lower contol arm (Autodesk Fusion 360 design; units mm, degrees)
Autodesk Fusion 360 part; units mm, degrees
sketch "Sketch1" plane through (0, -20.5, 43.25) normal (0, 0, 1) x (-1, 0, 0)
  arc A0 (2.75, -18.25) -> (2.25, -17.75) centre (2.25, -18.25) ccw
  line L0 (2.25, -17.75) -> (-2.25, -17.75)
  arc A1 (-2.25, -17.75) -> (-2.75, -18.25) centre (-2.25, -18.25) ccw
  line L1 (-2.75, -18.25) -> (-2.75, -22.75)
  arc A2 (-2.75, -22.75) -> (-2.25, -23.25) centre (-2.25, -22.75) ccw
  line L2 (-2.25, -23.25) -> (2.25, -23.25)
  arc A3 (2.25, -23.25) -> (2.75, -22.75) centre (2.25, -22.75) ccw
  line L3 (2.75, -22.75) -> (2.75, -18.25)
  line L4 (2.85, -22.75) -> (2.85, -18.25)
  arc A4 (2.85, -18.25) -> (2.25, -17.65) centre (2.25, -18.25) ccw
  line L5 (2.25, -17.65) -> (-2.25, -17.65)
  arc A5 (-2.25, -17.65) -> (-2.85, -18.25) centre (-2.25, -18.25) ccw
  line L6 (-2.85, -18.25) -> (-2.85, -22.75)
  arc A6 (-2.85, -22.75) -> (-2.25, -23.35) centre (-2.25, -22.75) ccw
  line L7 (-2.25, -23.35) -> (2.25, -23.35)
  arc A7 (2.25, -23.35) -> (2.85, -22.75) centre (2.25, -22.75) ccw
  circle A8 centre (0, -20.5) radius 3.95 construction
  circle A9 centre (0, -20.5) radius 6
  line L8 (0, -20.5) -> (-20, -20.5) construction
  circle A10 centre (-20, -20.5) radius 5
  line L9 (-0.3, -26.4925) -> (-20.25, -25.4937)
  line L10 (-0.3, -14.5075) -> (-20.25, -15.5063)
  dimension "d163" = 0.1
  dimension "d164" = 12
  dimension "d165" = 20
  dimension "d166" = 10
  constraint concentric A8 A9
  constraint coincident A8.centre A9.centre
  constraint perpendicular L6 L8
  constraint coincident L8.end A10.centre
  constraint coincident A9 L9.start
  constraint coincident A10 L9.end
  constraint tangent A10 L9
  constraint coincident A9 L10.start
  constraint coincident A10 L10.end
  constraint tangent A10 L10
  constraint tangent A9 L9
  constraint tangent A9 L10
  measures "d164" diameter of A9
  measures "d165" distance of A8.centre L8.end
  measures "d166" diameter of A10
extrude "Extrude1" add sketch "Sketch1" against normal blind 4 contours A9 | A9 A10 L9 L10 | A10 makes body 1
sketch "Sketch2" plane through (0, 0, 43.25) normal (0, 0, 1) x (-1, 0, 0)
  arc A0 (2.25, -2.85) -> (2.85, -2.25) centre (2.25, -2.25) ccw
  line L0 (2.25, -2.85) -> (-2.25, -2.85)
  arc A1 (-2.85, -2.25) -> (-2.25, -2.85) centre (-2.25, -2.25) ccw
  line L1 (-2.85, -2.25) -> (-2.85, 2.25)
  arc A2 (-2.25, 2.85) -> (-2.85, 2.25) centre (-2.25, 2.25) ccw
  line L2 (-2.25, 2.85) -> (2.25, 2.85)
  arc A3 (2.85, 2.25) -> (2.25, 2.85) centre (2.25, 2.25) ccw
  line L3 (2.85, 2.25) -> (2.85, -2.25)
  arc A4 (-0.3, -5.9925) -> (-0.3, 5.9925) centre (0, 0) ccw
  line L4 (-0.3, 5.9925) -> (-20.25, 4.9937)
  arc A5 (-20.25, 4.9937) -> (-20.25, -4.9937) centre (-20, 0) ccw
  line L5 (-20.25, -4.9937) -> (-0.3, -5.9925)
  circle A6 centre (0, 0) radius 1.25
  dimension "d169" = 2.5
  constraint concentric A4 A6
  measures "d169" diameter of A6
extrude "Extrude2" add sketch "Sketch2" along normal blind 1 contours A0 L0 A1 L1 A2 L2 A3 L3 | A4 L4 A5 L5 bodies 1
sketch "Sketch3" plane through (0, 0, 39.25) normal (0, 0, -1) x (1, 0, 0)
  arc A0 (-2.85, -2.25) -> (-2.25, -2.85) centre (-2.25, -2.25) ccw
  line L0 (-2.85, -2.25) -> (-2.85, 2.25)
  arc A1 (-2.25, 2.85) -> (-2.85, 2.25) centre (-2.25, 2.25) ccw
  line L1 (-2.25, 2.85) -> (2.25, 2.85)
  arc A2 (2.85, 2.25) -> (2.25, 2.85) centre (2.25, 2.25) ccw
  line L2 (2.85, 2.25) -> (2.85, -2.25)
  arc A3 (2.25, -2.85) -> (2.85, -2.25) centre (2.25, -2.25) ccw
  line L3 (2.25, -2.85) -> (-2.25, -2.85)
  arc A4 (0.3, 5.9925) -> (0.3, -5.9925) centre (0, 0) ccw
  line L4 (0.3, -5.9925) -> (20.25, -4.9937)
  arc A5 (20.25, -4.9937) -> (20.25, 4.9937) centre (20, 0) ccw
  line L5 (20.25, 4.9937) -> (0.3, 5.9925)
  circle A6 centre (20, 0) radius 2.95
  dimension "d172" = 5.9
  constraint concentric A5 A6
  measures "d172" diameter of A6
extrude "Extrude3" add sketch "Sketch3" along normal blind 4 contours A6 bodies 1
extrude "Extrude4" cut 1 faces at (18.7011, 0.7122, 35.25) along direction (0, 0, 1) blind 4 on bodies 1 bodies 1
sketch "Sketch4" plane through (0, 0, 39.25) normal (0, 0, -1) x (1, 0, 0)
  arc A0 (-2.85, -2.25) -> (-2.25, -2.85) centre (-2.25, -2.25) ccw
  line L0 (-2.85, -2.25) -> (-2.85, 2.25)
  arc A1 (-2.25, 2.85) -> (-2.85, 2.25) centre (-2.25, 2.25) ccw
  line L1 (-2.25, 2.85) -> (2.25, 2.85)
  arc A2 (2.85, 2.25) -> (2.25, 2.85) centre (2.25, 2.25) ccw
  line L2 (2.85, 2.25) -> (2.85, -2.25)
  arc A3 (2.25, -2.85) -> (2.85, -2.25) centre (2.25, -2.25) ccw
  line L3 (2.25, -2.85) -> (-2.25, -2.85)
  arc A4 (0.3, 5.9925) -> (0.3, -5.9925) centre (0, 0) ccw
  line L4 (0.3, -5.9925) -> (20.25, -4.9937)
  arc A5 (20.25, -4.9937) -> (20.25, 4.9937) centre (20, 0) ccw
  line L5 (20.25, 4.9937) -> (0.3, 5.9925)
  circle A6 centre (20, 0) radius 1.25
  dimension "d225" = 2.5
  constraint concentric A5 A6
  measures "d225" diameter of A6
extrude "Extrude5" cut sketch "Sketch4" against normal blind 2 contours A6 bodies 1
extrude "Extrude6" cut 1 faces at (20.367, -0.2927, 41.25) along direction (0, 0, 1) blind 0.8 draft 45 on bodies 1 bodies 1
extrude "Extrude7" cut 1 faces at (19.4991, 0.6685, 42.05) along direction (0, 0, 1) up to surface (2.2 mm away) on bodies 1 bodies 1
sketch "Sketch5" plane through (0, 0, 39.25) normal (0, 0, -1) x (1, 0, 0)
  circle A0 centre (20, 0) radius 1.25
  arc A1 (-2.85, -2.25) -> (-2.25, -2.85) centre (-2.25, -2.25) ccw
  line L0 (-2.85, -2.25) -> (-2.85, 2.25)
  arc A2 (-2.25, 2.85) -> (-2.85, 2.25) centre (-2.25, 2.25) ccw
  line L1 (-2.25, 2.85) -> (2.25, 2.85)
  arc A3 (2.85, 2.25) -> (2.25, 2.85) centre (2.25, 2.25) ccw
  line L2 (2.85, 2.25) -> (2.85, -2.25)
  arc A4 (2.25, -2.85) -> (2.85, -2.25) centre (2.25, -2.25) ccw
  line L3 (2.25, -2.85) -> (-2.25, -2.85)
  arc A5 (0.3, 5.9925) -> (0.3, -5.9925) centre (0, 0) ccw
  line L4 (0.3, -5.9925) -> (20.25, -4.9937)
  arc A6 (20.25, -4.9937) -> (20.25, 4.9937) centre (20, 0) ccw
  line L5 (20.25, 4.9937) -> (0.3, 5.9925)
  circle A7 centre (20, 0) radius 2.95
  circle A8 centre (20, 0) radius 0.8
  dimension "d232" = 5.9
  dimension "d233" = 1.6
  constraint concentric A0 A7
  constraint concentric A7 A8
  measures "d232" diameter of A7
  measures "d233" diameter of A8
extrude "Extrude8" add sketch "Sketch5" along normal blind 2.5 separate body contours A0 | A7 makes body 2
extrude "Extrude9" add 1 faces at (22.2194, 0.1863, 36.75) along direction (0, 0, -1) up to surface (8 mm away) draft 45 on bodies 2 bodies 2
fillet "Fillet1" radius 0.3 1 edges at (9.791, -3.9597, 28.75) on bodies 2
copy_body "Body->Comp1" bodies 2 removing the originals makes body 3 in component "pivot"
sketch "Sketch1 (2)" plane through (0, 0, 28.75) normal (0, 0, -1) x (1, 0, 0) in component "pivot"
  circle A0 centre (20, 0) radius 10.2257
  circle A1 centre (20, 0) radius 0.8
  dimension "d240" = 1.6
  constraint concentric A0 A1
  measures "d240" diameter of A1
extrude "Extrude1'" cut sketch "Sketch1 (2)" against normal blind 4 contours A1 bodies 3 in component "pivot"
